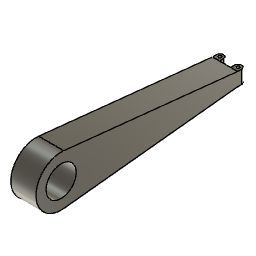
arm2 v3 (Autodesk Fusion 360 design; units mm, degrees)
Autodesk Fusion 360 part; units mm, degrees
sketch "Sketch1" plane through (0, 0, 0) normal (1, 0, 0) x (0, 1, 0)
  circle A0 centre (0, 0) radius 30
  line L0 (5.2264, 49.7261) -> (351.0282, 13.3809)
  line L1 (5.2991, -49.7184) -> (351.0282, -12.87)
  line L2 (351.0282, 13.3809) -> (351.0282, -12.87)
  arc A1 (5.2264, 49.7261) -> (5.2991, -49.7184) centre (0, 0) ccw
  dimension "d1" = 100
  dimension "d2" = 60
  constraint coincident A0.centre A1.centre
  constraint tangent L0 A1
  constraint vertical L2
  measures "d1" diameter of A1
  measures "d2" diameter of A0
extrude "Extrude1" add sketch "Sketch1" along normal blind 50
sketch "Sketch2" plane through (0, 0, 0) normal (0, 0, 1) x (1, 0, 0)
  line L0 (50, 351) -> (36, 351)
  line L1 (36, 351) -> (36, 359)
  line L2 (50, 359) -> (50, 351)
  circle A0 centre (43, 359) radius 3
  line L3 (0, 351) -> (14, 351)
  line L4 (14, 351) -> (14, 359)
  line L5 (0, 359) -> (0, 351)
  circle A1 centre (7, 359) radius 3
  arc A2 (50, 359) -> (36, 359) centre (43, 359) ccw
  arc A3 (14, 359) -> (0, 359) centre (7, 359) ccw
  dimension "d9" = 6
  dimension "d12" = 6
  constraint horizontal L0
  constraint vertical L1
  constraint vertical L2
  constraint concentric A0 A2
  constraint horizontal L3
  constraint vertical L4
  constraint vertical L5
  constraint concentric A1 A3
  measures "d9" diameter of A0
  measures "d12" diameter of A1
extrude "Extrude2" add sketch "Sketch2" along normal blind 13.355 and the other way blind 13.1255
equation "d13 = ( 26.71 / 2 ) * 1 mm"
equation "d15 = ( 26.251 / 2 ) * 1 mm"
